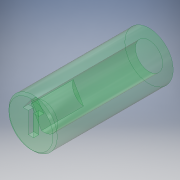
# Autodesk Inventor part: potcap
Saved by Autodesk Inventor 2017 SP1 (Build 210196100, 196)
## iProperties
Created: 2016-12-24
Part Number: potcap
Material: Generic
Document SubType Name: Modeling
Designer: wsh32
Density: 1 g/cm^3
Appearance: Clear - Green 1
Author: wsh32
Autodesk Inventor part; units mm, degrees
ref_plane "YZ Plane" through (0, 0, 0) normal (1, 0, 0) x (0, 1, 0)
ref_plane "XZ Plane" through (0, 0, 0) normal (0, 1, 0) x (-1, 0, 0)
ref_plane "XY Plane" through (0, 0, 0) normal (0, 0, 1) x (1, 0, 0)
sketch "Sketch1" plane through (0, 0, 0) normal (0, 0, 1) x (1, 0, 0)
  circle A0 centre (0, 0) radius 2.9845
  circle A1 centre (0, 0) radius 5.842
  circle A2 centre (0, 0) radius 3.302
  dimension "d0" = 5.969
  dimension "d2" = 0.3175
  dimension "d5" = 2.54
  constraints: 3 centre point, 1 coincident
  measures "d0" diameter of A0
  measures "d2" radial gap between concentric circles of A0 A2
  measures "d5" radial gap between concentric circles of A1 A2
extrude "Extrusion1" add sketch "Sketch1" along normal blind 25.4 contours A1
sketch "Sketch2" plane through (0, 0, 25.4) normal (0, 0, 1) x (1, 0, 0)
  circle A0 centre (0, 0) radius 5.842 projected
extrude "Extrusion2" add sketch "Sketch2" along normal blind 3.175
sketch "Sketch3" plane through (0, 0, 28.575) normal (0, 0, 1) x (1, 0, 0)
  line L0 (0.635, -2.54) -> (-0.635, -2.54)
  line L1 (-0.635, -2.54) -> (-0.635, 2.54)
  line L2 (-0.635, 2.54) -> (0.635, 2.54)
  line L3 (0.635, 2.54) -> (0.635, -2.54)
  line L4 (0.635, -2.54) -> (-0.635, 2.54) construction
  line L5 (-0.635, -2.54) -> (0.635, 2.54) construction
  line L6 (0, 2.54) -> (0, -2.54) construction
  line L7 (-1.905, 2.54) -> (1.905, 2.54)
  line L8 (1.905, 2.54) -> (0, 5.08)
  line L9 (0, 5.08) -> (-1.905, 2.54)
  point P0 (0, 0)
  dimension "d8" = 5.08
  dimension "d9" = 2.54
  dimension "d10" = 1.27
  dimension "d11" = 3.81
  constraints: 20 end point, 4 midpoint, 2 horizontal, 2 parallel, 1 collinear, 1 perpendicular, 1 point on line, 1 symmetric about line
  measures "d8" distance of L2.end L0.start
  measures "d9" distance from line of L8.end L7
  measures "d10" distance of L1.end L2.end
  measures "d11" distance of L7.start L7.end
extrude "Extrusion3" cut sketch "Sketch3" against normal blind 1.27
chamfer "Chamfer1" distance 0.508 angle 45 1 edges at (-5.842, 0, 28.575)
sketch "Sketch6" plane through (0, 0, 25.4) normal (0, 0, -1) x (-1, 0, 0)
  circle A0 centre (0, 0) radius 3.302 projected
  line L0 (0.6206, 3.2432) -> (3.1189, -1.0842) construction
  line L1 (3.1189, 1.0842) -> (0.6206, -3.2432)
  line L2 (0, 0) -> (3.302, 0) construction
  circle A1 centre (0, 0) radius 3.302 construction
  line L3 (0, 0) -> (2.8596, -1.651) construction
  line L4 (0, 0) -> (2.8596, 1.651) construction
  line L5 (-1.3144, 4.3273) -> (-3.8128, 0) construction
  arc A2 (0.6206, -3.2432) -> (3.1189, 1.0842) centre (0, 0) ccw
  dimension "d24" = 60
  dimension "d26" = 5.461
  constraints: 12 end point, 4 point on circle, 2 equal length, 2 symmetric about line, 1 centre point, 1 horizontal, 1 parallel, 1 point on line, 11 other
  measures "d24" angle of L3 L4
  measures "d26" distance between parallel lines of L5 L1
extrude "Extrusion6" add sketch "Sketch6" along normal blind 10.16 contours A0 L1 picked at (1.6947, -1.725)
equation "\"d9\" = 0.5 * d8"
equation "\"d11\" = 3 * d10"
body "Solid1"
